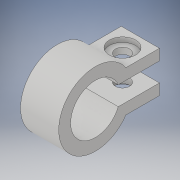
# Autodesk Inventor part: 10mm rod Top Clamp
Saved by Autodesk Inventor 2019 (Build 230136000, 136)
## iProperties
Created: 2019-07-23
Part Number: 10mm rod Top Clamp
Material: Generic
Document SubType Name: Modeling
Designer: Matthew XPS
Density: 1 g/cm^3
Appearance: Default
Author: Matthew XPS
Autodesk Inventor part; units mm, degrees
ref_plane "YZ Plane" through (0, 0, 0) normal (1, 0, 0) x (0, 1, 0)
ref_plane "XZ Plane" through (0, 0, 0) normal (0, 1, 0) x (-1, 0, 0)
ref_plane "XY Plane" through (0, 0, 0) normal (0, 0, 1) x (1, 0, 0)
sketch "Sketch2" plane through (0, 0, 0) normal (1, 0, 0) x (0, 1, 0)
  arc A0 (2, -4.8) -> (-2, -4.8) centre (0, 0) ccw
  arc A1 (2, -7.4357) -> (-2, -7.4357) centre (0, 0) ccw
  line L0 (0, 0) -> (2, -4.8)
  line L1 (2, -4.8) -> (2, -7.4357)
  line L2 (2, -7.4357) -> (2, -13.4357)
  line L3 (2, -13.4357) -> (4.3, -13.4357)
  line L4 (4.3, -13.4357) -> (4.3, -6.3875)
  line L5 (0, 0) -> (0, -16.8496) construction
  line L6 (0, 0) -> (-2, -4.8)
  line L7 (-2, -4.8) -> (-2, -7.4357)
  line L8 (-2, -7.4357) -> (-2, -13.4357)
  line L9 (-2, -13.4357) -> (-4.3, -13.4357)
  line L10 (-4.3, -13.4357) -> (-4.3, -6.3875)
  line L11 (-4.3, -6.3875) -> (-2, -6.3875)
  arc A2 (0, -5.2) -> (2, -4.8) centre (0, 0) ccw
  arc A3 (0, -7.7) -> (2, -7.4357) centre (0, 0) ccw
  arc A4 (-2, -7.4357) -> (0, -7.7) centre (0, 0) ccw
  arc A5 (-2, -4.8) -> (0, -5.2) centre (0, 0) ccw
  dimension "d6" = 10.4
  dimension "d7" = 2.5
  dimension "d9" = 2
  dimension "d10" = 6
  dimension "d11" = 2.3
  dimension "d12" = 90
  constraints: 24 end point, 14 point on circle, 6 centre point, 5 point on line, 5 symmetric about line, 2 perpendicular, 2 vertical, 1 coincident, 1 horizontal
  measures "d6" diameter of A0
  measures "d7" radial gap between concentric circles of A0 A1
  measures "d9" horizontal distance of point (0, 0) L0.end
  measures "d10" distance of L1.end L2.end
  measures "d11" distance of L2.end L3.end
  measures "d12" angle of L3 L2
extrude "Extrusion1" add sketch "Sketch2" along normal blind 8 contours A0 L7 L11 A1 L1 | A1 L4 L3 L2 | L7 A1 L11 | L8 L9 L10 A1
sketch "Sketch3" plane through (0, 4.3, -6.3875) normal (0, 1, 0) x (1, 0, 0)
  line L0 (0, 7.0482) -> (0, 0) projected
  line L1 (0, 0) -> (8, 0) projected
  line L2 (8, 7.0482) -> (8, 0) projected
  line L3 (0, 7.0482) -> (8, 7.0482) projected
  circle A0 centre (4, 3.3) radius 1.5
  point P0 (0, -6.3875)
  dimension "d15" = 3
  dimension "d21" = 3.3
  constraints: 1 centre point
  measures "d15" diameter of A0
  measures "d21" distance from line of L1 A0.centre
extrude "Extrusion2" cut sketch "Sketch3" against normal up to next contours A0
sketch "Sketch4" plane through (0, 4.3, -6.3875) normal (0, 1, 0) x (1, 0, 0)
  line L0 (0, 7.0482) -> (0, -1.5875) projected
  line L1 (0, -1.5875) -> (8, -1.5875) projected
  line L2 (8, 7.0482) -> (8, -1.5875) projected
  line L3 (0, 7.0482) -> (8, 7.0482) projected
  circle A0 centre (4, 3.3) radius 1.5 projected
  line L4 (0, 7.0482) -> (0, 0) projected
  line L5 (0, 0) -> (8, 0) projected
  line L6 (8, 7.0482) -> (8, 0) projected
  line L7 (0, 7.0482) -> (8, 7.0482) projected
  circle A1 centre (4, 3.3) radius 2.75
  point P0 (0, -6.3875)
  dimension "d18" = 5.5
  constraints: 1 centre point, 1 coincident
  measures "d18" diameter of A1
extrude "Extrusion3" cut sketch "Sketch4" against normal blind 1 contours A1
mirror "Mirror1" about plane through (0, 0, 0) normal (0, 1, 0) of "Extrusion3", "Extrusion2"
body "Solid1"
